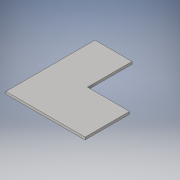
# Autodesk Inventor part: RSX top
Saved by Autodesk Inventor 2016 (Build 200138000, 138)
## iProperties
Created: 2017-04-05
Part Number: RSX top
Material: Generic
Document SubType Name: Modeling
Designer: Ethan
Density: 1 g/cm^3
Appearance: Default
Author: Ethan
Autodesk Inventor part; units mm, degrees
ref_plane "YZ Plane" through (0, 0, 0) normal (1, 0, 0) x (0, 1, 0)
ref_plane "XZ Plane" through (0, 0, 0) normal (0, 1, 0) x (-1, 0, 0)
ref_plane "XY Plane" through (0, 0, 0) normal (0, 0, 1) x (1, 0, 0)
sketch "Sketch1" plane through (0, 0, 0) normal (0, 1, 0) x (-1, 0, 0)
  point P0 (0, 0)
sketch "Sketch2" plane through (0, 0, 0) normal (0, 1, 0) x (-1, 0, 0)
  line L0 (0, 0) -> (177.8, 0)
  line L1 (177.8, 0) -> (177.8, -203.2)
  line L2 (0, 0) -> (0, -88.9)
  line L3 (177.8, -203.2) -> (107.95, -203.2)
  line L4 (107.95, -203.2) -> (107.95, -88.9)
  line L5 (0, -88.9) -> (107.95, -88.9)
  line L6 (190.5, -215.9) -> (190.5, 12.7)
  line L7 (190.5, 12.7) -> (-12.7, 12.7)
  line L8 (-12.7, 12.7) -> (-12.7, -101.6)
  line L9 (-12.7, -101.6) -> (95.25, -101.6)
  line L10 (95.25, -101.6) -> (95.25, -215.9)
  line L11 (95.25, -215.9) -> (190.5, -215.9)
  dimension "d0" = 203.2
  dimension "d1" = 177.8
  dimension "d2" = 88.9
  dimension "d3" = 69.85
  dimension "d4" = 12.7
  constraints: 24 end point, 3 horizontal, 2 perpendicular, 1 vertical, 5 other
  measures "d0" distance of L0.end L1.end
  measures "d1" distance of L0.start L0.end
  measures "d2" distance of L0.start L2.end
  measures "d3" distance of L1.end L3.end
  measures "d4" distance between parallel lines of L1 L6
extrude "Extrusion1" add sketch "Sketch2" along normal blind 6.35 contours L0 L1 L3 L4 L5 L2 | L11 L10 L9 L8 L7 L6
body "Solid1"
